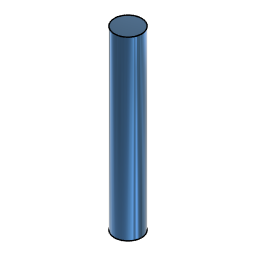
UV Box Model v29 (Autodesk Fusion 360 archive; units mm, degrees)
design "tube"
Autodesk Fusion 360 part; units mm, degrees
cylinder "CylinderPrimitive1" add diameter 20 height 130 placed x (1, 0, 0) y (0, 1, 0) z (0, 0, 1) at (0, 0, 0)

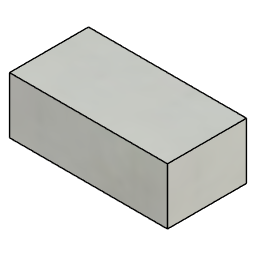
design "light"
Autodesk Fusion 360 part; units mm, degrees
sketch "Sketch1" plane through (0, 0, 0) normal (0, 0, 1) x (1, 0, 0)
  line L0 (0, 0) -> (14, 0)
  line L1 (14, 0) -> (14, -7)
  line L2 (14, -7) -> (0, -7)
  line L3 (0, -7) -> (0, 0)
  dimension "d1" = 14
  dimension "d2" = 7
  constraint horizontal L0
  constraint vertical L1
  constraint horizontal L2
  constraint vertical L3
  constraint coincident L0.start L3.end
  measures "d1" distance of L0.start L0.end
  measures "d2" distance of L0.start L2.end
extrude "Extrude1" add sketch "Sketch1" along normal blind 5

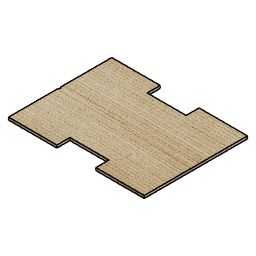
design "inner"
Autodesk Fusion 360 part; units mm, degrees
sketch "Sketch1" plane through (0, 0, 0) normal (0, 0, 1) x (1, 0, 0)
  line L0 (209, -159) -> (-209, -159)
  line L1 (-209, -159) -> (-209, 159)
  line L2 (-209, 159) -> (209, 159)
  line L3 (209, 159) -> (209, -159)
  line L4 (209, -159) -> (-209, 159) construction
  line L5 (-209, -159) -> (209, 159) construction
  line L6 (60, 119) -> (-60, 119)
  line L7 (-60, 119) -> (-60, 199)
  line L8 (-60, 199) -> (60, 199)
  line L9 (60, 199) -> (60, 119)
  line L10 (60, 119) -> (-60, 199) construction
  line L11 (-60, 119) -> (60, 199) construction
  line L12 (60, -119) -> (-60, -119)
  line L13 (-60, -119) -> (-60, -199)
  line L14 (-60, -199) -> (60, -199)
  line L15 (60, -199) -> (60, -119)
  line L16 (60, -119) -> (-60, -199) construction
  line L17 (-60, -119) -> (60, -199) construction
  point P0 (0, 159)
  point P1 (0, -159)
  dimension "d1" = 418
  dimension "d2" = 318
  dimension "d3" = 80
  dimension "d4" = 120
  dimension "d5" = 80
  constraint horizontal L0
  constraint perpendicular L0 L1
  constraint parallel L0 L2
  constraint parallel L1 L3
  constraint coincident L4 origin
  constraint coincident L5 origin
  constraint horizontal L6
  constraint perpendicular L6 L7
  constraint parallel L6 L8
  constraint parallel L7 L9
  constraint coincident L10 P0
  constraint coincident L11 P0
  constraint midpoint L2 P0
  constraint horizontal L12
  constraint perpendicular L12 L13
  constraint parallel L12 L14
  constraint parallel L13 L15
  constraint coincident L16 P1
  constraint coincident L17 P1
  constraint midpoint L0 P1
  measures "d1" distance of L1.end L2.end
  measures "d2" distance of L0.end L1.end
  measures "d3" distance of L6.end L7.end
  measures "d4" distance of L13.end L14.end
  measures "d5" distance of L12.end L13.end
extrude "Extrude1" add sketch "Sketch1" along normal blind 8 contours L0 L1 L2 L3 L6 L7 L9 L12 L13 L15
sketch "Sketch2" plane through (0, 0, 8) normal (0, 0, 1) x (-1, 0, 0)
  line L0 (-60, -159) -> (-60, -119)
  line L1 (-60, -119) -> (60, -119)
  line L2 (60, -119) -> (60, -159)
  line L3 (60, -159) -> (209, -159)
  line L4 (209, -159) -> (209, 159)
  line L5 (209, 159) -> (60, 159)
  line L6 (60, 159) -> (60, 119)
  line L7 (60, 119) -> (-60, 119)
  line L8 (-60, 119) -> (-60, 159)
  line L9 (-60, 159) -> (-209, 159)
  line L10 (-209, 159) -> (-209, -159)
  line L11 (-209, -159) -> (-60, -159)
  line L12 (209, 0) -> (206, 0)
  line L13 (206, 0) -> (206, 6)
  line L14 (206, 6) -> (209, 6)
  line L15 (209, 6) -> (209, 0)
  line L16 (209, 0) -> (206, 0)
  line L17 (206, 0) -> (206, 6)
  line L18 (206, 6) -> (209, 6)
  line L19 (209, 6) -> (209, 0)
  dimension "d8" = 3
  dimension "d9" = 6
  dimension "d10" = 6
  constraint horizontal L12
  constraint vertical L13
  constraint horizontal L14
  constraint vertical L15
  constraint midpoint L4 L12.start
  constraint horizontal L16
  constraint vertical L17
  constraint horizontal L18
  constraint vertical L19
  measures "d8" distance of L12.start L12.end
  measures "d9" distance of L12.start L14.end
  measures "d10" distance of L12.start L14.end
extrude "Extrude2" cut sketch "Sketch2" against normal blind 13 contours L4 L12 L13 L14 L15 L16 L17 L18 L19
equation "d1 = 450 mm - ( 2 * 16 ) * 1 mm"
equation "d2 = 350 mm - ( 2 * 16 ) * 1 mm"

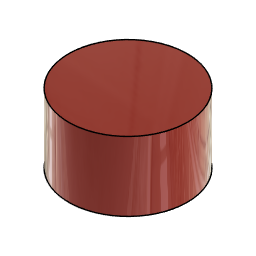
design "button"
Autodesk Fusion 360 part; units mm, degrees
sketch "Sketch1" plane through (0, 0, 0) normal (0, 0, 1) x (1, 0, 0)
  circle A0 centre (0, 0) radius 6
  dimension "d1" = 12
  constraint coincident A0.centre origin
  measures "d1" diameter of A0
extrude "Extrude1" add sketch "Sketch1" along normal blind 7
